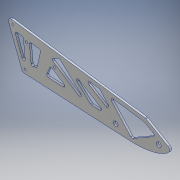
# Autodesk Inventor part: bracket1
Saved by Autodesk Inventor 2018 (Build 220112000, 112)
## iProperties
Created: 2018-03-05
Part Number: bracket1
Material: アルミニウム 6061
Document SubType Name: Modeling
Designer: ku_sk
Density: 2.7 g/cm^3
Appearance: アルミニウム - フラット
Mass: 456.161 g
Surface Area: 733.858 cm^2
Volume: 168.949 cm^3
Author: ku_sk
Autodesk Inventor part; units mm, degrees
ref_plane "YZ Plane" through (0, 0, 0) normal (1, 0, 0) x (0, 1, 0)
ref_plane "XZ Plane" through (0, 0, 0) normal (0, 1, 0) x (-1, 0, 0)
ref_plane "XY Plane" through (0, 0, 0) normal (0, 0, 1) x (1, 0, 0)
sketch "スケッチ2" plane through (0, 0, 0) normal (0, 1, 0) x (-1, 0, 0)
  arc A0 (320.7468, 34.8983) -> (392.1215, 71.6787) centre (243.1623, 273.099) ccw projected
  arc A1 (310.5095, 31.8959) -> (320.7468, 34.8983) centre (264.9264, 206.2785) ccw projected
  arc A2 (290.9118, 29.5172) -> (310.5095, 31.8959) centre (291.9468, 102.9093) ccw projected
  arc A3 (278.6891, 31.4878) -> (290.9118, 29.5172) centre (291.5128, 72.1352) ccw projected
  arc A4 (274.9831, 33.389) -> (278.6891, 31.4878) centre (282.4278, 43.3382) ccw projected
  arc A5 (275.4733, 39.2078) -> (274.9831, 33.389) centre (277.0456, 36.1453) ccw projected
  arc A6 (283.1253, 42.3274) -> (275.4733, 39.2078) centre (297.1464, -3.0086) ccw projected
  arc A7 (310.1184, 49.282) -> (283.1253, 42.3274) centre (369.3413, -236.446) ccw projected
  arc A8 (310.1184, 49.282) -> (326.9533, 52.7997) centre (-771.7798, 5269.0252) ccw projected
  arc A9 (326.9533, 52.7997) -> (357.98, 60.8795) centre (256.8539, 385.5961) ccw projected
  arc A10 (357.98, 60.8795) -> (391.1188, 73.3957) centre (268.9975, 346.6028) ccw projected
  arc A11 (392.1215, 71.6787) -> (391.1188, 73.3957) centre (391.5269, 72.4828) ccw projected
  circle A12 centre (287.1934, 37.1564) radius 3 projected
  circle A13 centre (359.7933, 56.2153) radius 3 projected
  arc A14 (100.5026, -29.4375) -> (303.8176, 17.6729) centre (68.6386, 570.3585) ccw projected
  arc A15 (74.9408, -30.0377) -> (100.5026, -29.4375) centre (77.5861, 401.9345) ccw projected
  arc A16 (28.1912, -23.4013) -> (74.9408, -30.0377) centre (76.0159, 145.5175) ccw projected
  arc A17 (1.2395, -11.312) -> (28.1912, -23.4013) centre (55.8939, 74.446) ccw projected
  arc A18 (-6.0217, -4.7376) -> (1.2395, -11.312) centre (16.9451, 13.3315) ccw projected
  arc A19 (-1.6159, 7.4897) -> (-6.0217, -4.7376) centre (0, 0) ccw projected
  arc A20 (17.9572, 9.9554) -> (-1.6159, 7.4897) centre (22.277, -103.2534) ccw projected
  arc A21 (84.7958, 9.311) -> (17.9572, 9.9554) centre (44.6377, -689.2581) ccw projected
  arc A22 (84.7958, 9.311) -> (126.0099, 7.0084) centre (819.0754, 12782.4716) ccw projected
  arc A23 (126.0099, 7.0084) -> (203.0122, 6.466) centre (170.258, 822.6468) ccw projected
  arc A24 (203.0122, 6.466) -> (303.8176, 17.6729) centre (174.1884, 724.7085) ccw projected
  circle A25 centre (20.0666, -1.5588) radius 5 projected
  circle A26 centre (130.4331, -10.1322) radius 5 projected
  line L0 (100.5026, -29.4375) -> (370, -15.1205)
  line L1 (-3.831, 6.6355) -> (54.1787, 40.1274)
  line L2 (1137.2465, 0) -> (-1089.9509, 0) projected
  line L3 (54.1787, 40.1274) -> (410, 89.8795)
  line L4 (370, -15.1205) -> (410, 89.8795)
  point P0 (0, 0)
  point P1 (371.2778, 57.8193)
  dimension "d7" = 30
  dimension "d115" = 370
  dimension "d164" = 40
  dimension "d165" = 105
  constraints: 8 end point, 2 point on circle, 2 tangent
  measures "d7" angle of L2 L1
  measures "d115" horizontal distance of L0.end point (0, 0)
  measures "d164" horizontal distance of L3.end L0.end
  measures "d165" vertical distance of L0.end L3.end
extrude "押し出し3" add sketch "スケッチ2" along normal blind 5 contours A1 A2 A3 A4 A5 A6 A7 A8 A9 A10 A11 A0 | A15 A16 A17 A18 A19 L2 A25 A14 | A14 L2 L4 L0 | L2 A25 A19 A20 A21 A22 A23 A24 A14 | A14 A24 A23 A22 A21 A20 A19 L1 L3 L4 L2
fillet "フィレット2" radius 6 2 edges at (-54.1787, 2.5, 40.1274) (-370, 2.5, -15.1205)
fillet "フィレット2" radius 7 1 edges at (-410, 2.5, 89.8795)
sketch "スケッチ4" plane through (0, 5, 0) normal (0, 1, 0) x (1, 0, 0)
  circle A0 centre (-362.9716, 5.4798) radius 2.5
  line L0 (-53.1667, -39.5431) -> (3.831, -6.6355) projected
  line L1 (-410, -89.8795) -> (-55.3359, -40.2892) projected
  line L2 (-100.5026, 29.4375) -> (-366.1013, 15.3276) projected
  line L3 (-371.3899, 11.472) -> (-410, -89.8795) projected
  circle A1 centre (-394.6339, -77.6337) radius 2.5
  point P0 (0, 0)
  dimension "d21" = 5
  dimension "d22" = 10
  dimension "d23" = 10
  dimension "d77" = 10
  dimension "d78" = 10
  dimension "d79" = 5
  constraints: 2 centre point
  measures "d21" diameter of A0
  measures "d22" distance from line of L2 A0.centre
  measures "d23" distance from line of L3 A0.centre
  measures "d77" distance from line of A1.centre L1
  measures "d78" distance from line of L3 A1.centre
  measures "d79" diameter of A1
sketch "スケッチ6" plane through (0, 0, 0) normal (0, -1, 0) x (1, 0, 0)
  circle A0 centre (-20.0666, -1.5588) radius 6
  circle A1 centre (-20.0666, -1.5588) radius 5 projected
  circle A2 centre (-130.4331, -10.1322) radius 6
  circle A3 centre (-130.4331, -10.1322) radius 5 projected
  point P0 (0, 0)
  dimension "d29" = 12
  dimension "d30" = 12
  constraints: 2 centre point, 2 concentric
  measures "d29" diameter of A0
  measures "d30" diameter of A2
extrude "押し出し7" cut sketch "スケッチ6" against normal through all
extrude "押し出し9" cut sketch "スケッチ4" against normal through all
sketch "スケッチ10" plane through (0, 0, 0) normal (0, -1, 0) x (1, 0, 0)
  line L0 (-224.8903, 4.737) -> (-291.6748, 48.1758)
  line L1 (-291.3072, 55.0942) -> (-278.1848, 61.7685)
  line L2 (-273.6413, 61.1266) -> (-219.9793, 11.0136)
  line L3 (-195.2115, 1.5663) -> (-230.0713, 34.1207)
  line L4 (-225.2835, 40.4742) -> (-169.1321, 6.7888)
  line L5 (-171.402, -0.6357) -> (-192.6936, 0.4954)
  line L6 (-265.5172, 4.3641) -> (-303.9103, 6.4038)
  line L7 (-307.379, 11.9637) -> (-299.7389, 29.9268)
  line L8 (-293.877, 31.7143) -> (-263.1241, 11.7116)
  line L9 (-370.8987, 15.329) -> (-388.1624, 60.646)
  line L10 (-383.8705, 66.0314) -> (-371.07, 64.2416)
  line L11 (-367.6448, 60.6882) -> (-363.1817, 17.161)
  line L12 (-197.0925, 50.0128) -> (-173.4392, 46.7055)
  line L13 (-171.0224, 45.4227) -> (-149.6481, 21.7177)
  line L14 (-154.6766, 15.609) -> (-199.7042, 42.6212)
  line L15 (-347.6131, 60.9618) -> (-327.0753, 58.0901)
  line L16 (-323.7311, 53.2316) -> (-332.2966, 16.0111)
  line L17 (-335.1019, 13.0603) -> (-342.7409, 10.8908)
  line L18 (-347.8128, 14.3307) -> (-352.1462, 56.5923)
  line L19 (-138.0022, 41.7506) -> (-58.2636, 30.6013)
  line L20 (-56.8175, 30.1039) -> (-33.4921, 16.637)
  line L21 (-33.4921, 9.7088) -> (-86.6743, -20.996)
  line L22 (-91.645, -20.2105) -> (-141.5268, 35.1105)
  line L23 (-53.1667, 39.5431) -> (3.831, 6.6355) projected
  line L24 (-398.2744, 88.24) -> (-55.3359, 40.2892) projected
  line L25 (-371.3899, -11.472) -> (-405.7851, 78.8155) projected
  circle A0 centre (-362.9716, -5.4798) radius 2.5 projected
  circle A1 centre (-394.6339, 77.6337) radius 2.5 projected
  circle A2 centre (-20.0666, -1.5588) radius 6 projected
  circle A3 centre (-130.4331, -10.1322) radius 6 projected
  arc A4 (-398.2744, 88.24) -> (-405.7851, 78.8155) centre (-399.2437, 81.3074) ccw projected
  line L26 (-371.3899, -11.472) -> (-405.7851, 78.8155) projected
  arc A5 (-371.3899, -11.472) -> (-366.1013, -15.3276) centre (-365.783, -9.3361) ccw projected
  line L27 (-100.5026, -29.4375) -> (-366.1013, -15.3276) projected
  arc A6 (-100.5026, -29.4375) -> (-74.9408, -30.0377) centre (-77.5861, 401.9345) ccw projected
  arc A7 (-74.9408, -30.0377) -> (-28.1912, -23.4013) centre (-76.0159, 145.5175) ccw projected
  arc A8 (-28.1912, -23.4013) -> (-1.2395, -11.312) centre (-55.8939, 74.446) ccw projected
  arc A9 (-1.2395, -11.312) -> (6.0217, -4.7376) centre (-16.9451, 13.3315) ccw projected
  arc A10 (6.0217, -4.7376) -> (3.831, 6.6355) centre (0, 0) ccw projected
  line L28 (-53.1667, 39.5431) -> (3.831, 6.6355) projected
  arc A11 (-53.1667, 39.5431) -> (-55.3359, 40.2892) centre (-56.1667, 34.347) ccw projected
  line L29 (-398.2744, 88.24) -> (-55.3359, 40.2892) projected
  circle A12 centre (-287.1934, 37.1564) radius 3 projected
  circle A13 centre (-359.7933, 56.2153) radius 3 projected
  arc A14 (-370.8987, 15.329) -> (-363.1817, 17.161) centre (-367.1608, 16.7529) ccw
  arc A15 (-383.8705, 66.0314) -> (-388.1624, 60.646) centre (-384.4244, 62.07) ccw
  arc A16 (-367.6448, 60.6882) -> (-371.07, 64.2416) centre (-371.6239, 60.2802) ccw
  arc A17 (-347.6131, 60.9618) -> (-352.1462, 56.5923) centre (-348.167, 57.0004) ccw
  arc A18 (-347.8128, 14.3307) -> (-342.7409, 10.8908) centre (-343.8337, 14.7387) ccw
  arc A19 (-335.1019, 13.0603) -> (-332.2966, 16.0111) centre (-336.1947, 16.9081) ccw
  arc A20 (-323.7311, 53.2316) -> (-327.0753, 58.0901) centre (-327.6292, 54.1287) ccw
  arc A21 (-293.877, 31.7143) -> (-299.7389, 29.9268) centre (-296.058, 28.3612) ccw
  arc A22 (-307.379, 11.9637) -> (-303.9103, 6.4038) centre (-303.6981, 10.3981) ccw
  arc A23 (-265.5172, 4.3641) -> (-263.1241, 11.7116) centre (-265.305, 8.3585) ccw
  arc A24 (-291.3072, 55.0942) -> (-291.6748, 48.1758) centre (-289.4938, 51.5289) ccw
  arc A25 (-273.6413, 61.1266) -> (-278.1848, 61.7685) centre (-276.3714, 58.2031) ccw
  arc A26 (-224.8903, 4.737) -> (-219.9793, 11.0136) centre (-222.7094, 8.0901) ccw
  arc A27 (-225.2835, 40.4742) -> (-230.0713, 34.1207) centre (-227.3412, 37.0441) ccw
  arc A28 (-171.402, -0.6357) -> (-169.1321, 6.7888) centre (-171.1898, 3.3587) ccw
  arc A29 (-195.2115, 1.5663) -> (-192.6936, 0.4954) centre (-192.4814, 4.4898) ccw
  arc A30 (-197.0925, 50.0128) -> (-199.7042, 42.6212) centre (-197.6465, 46.0513) ccw
  arc A31 (-171.0224, 45.4227) -> (-173.4392, 46.7055) centre (-173.9931, 42.744) ccw
  arc A32 (-154.6766, 15.609) -> (-149.6481, 21.7177) centre (-152.6188, 19.0391) ccw
  arc A33 (-138.0022, 41.7506) -> (-141.5268, 35.1105) centre (-138.5561, 37.7891) ccw
  arc A34 (-91.645, -20.2105) -> (-86.6743, -20.996) centre (-88.6743, -17.5319) ccw
  arc A35 (-33.4921, 9.7088) -> (-33.4921, 16.637) centre (-35.4921, 13.1729) ccw
  arc A36 (-56.8175, 30.1039) -> (-58.2636, 30.6013) centre (-58.8175, 26.6398) ccw
  point P0 (0, 0)
  point P1 (-186.5641, -20.1916)
  point P2 (-297.4825, 51.9533)
  point P3 (-275.6884, 63.0382)
  point P4 (-194.1474, 0.5726)
  point P5 (-257.6969, 59.9191)
  point P6 (-155.3329, -1.4894)
  point P7 (-250.6102, 3.5722)
  point P8 (-309.6149, 6.7068)
  point P9 (-297.8731, 34.3135)
  point P10 (-360.0825, -13.0636)
  point P11 (-390.5709, 66.9683)
  point P12 (-367.9646, 63.8074)
  point P13 (-216.5638, 52.7353)
  point P14 (-171.9973, 46.5039)
  point P15 (-131.7251, 1.8403)
  point P16 (-352.6667, 61.6684)
  point P17 (-322.7521, 57.4857)
  point P18 (-332.8269, 13.7064)
  point P19 (-347.3266, 9.5885)
  point P20 (-148.8863, 43.2724)
  point P21 (-57.4921, 30.4934)
  point P22 (-27.4921, 13.1729)
  point P23 (-89.4775, -22.6144)
  dimension "d194" = 10
  dimension "d196" = 10
  dimension "d197" = 20
  dimension "d198" = 10
  dimension "d199" = 60
  dimension "d200" = 40
  dimension "d201" = 30
  dimension "d202" = 70
  dimension "d203" = 15
  dimension "d204" = 15
  dimension "d205" = 10
  dimension "d206" = 15
  dimension "d207" = 15
  dimension "d209" = 25
  dimension "d210" = 15
  dimension "d213" = 80
  dimension "d214" = 85
  dimension "d216" = 70
  dimension "d218" = 45
  dimension "d219" = 70
  dimension "d222" = 30
  dimension "d224" = 85
  dimension "d225" = 30
  dimension "d226" = 30
  dimension "d227" = 60
  dimension "d231" = 110
  dimension "d237" = 23
  dimension "d238" = 45
  dimension "d240" = 4
  constraints: 46 end point, 46 point on circle, 46 point on line, 46 tangent, 23 centre point, 22 equal radius, 11 parallel, 3 collinear
  measures "d194" distance between parallel lines of L23 L20
  measures "d196" distance between parallel lines of L24 L19
  measures "d197" distance between parallel lines of L24 L15
  measures "d198" distance between parallel lines of L25 L9
  measures "d199" angle of L21 L20
  measures "d200" angle of L22 L19
  measures "d201" distance from line of point (-57.492, 30.493) L21
  measures "d202" distance from line of point (-27.492, 13.173) L22
  measures "d203" distance between parallel lines of L22 L13
  measures "d204" distance between parallel lines of L4 L14
  measures "d205" distance between parallel lines of L2 L3
  measures "d206" angle of L9 L11
  measures "d207" distance between parallel lines of L8 L0
  measures "d209" distance between parallel lines of L27 L6
  measures "d210" distance between parallel lines of L18 L11
  measures "d213" angle of L18 L17
  measures "d214" angle of L16 L15
  measures "d216" distance from line of L26 point (-322.752, 57.486)
  measures "d218" distance from line of L25 point (-332.827, 13.706)
  measures "d219" angle of L6 L7
  measures "d222" angle of L6 L8
  measures "d224" distance from line of L25 point (-297.873, 34.314)
  measures "d225" distance of point (-309.615, 6.707) point (-297.873, 34.314)
  measures "d226" distance from line of L26 point (-367.965, 63.807)
  measures "d227" angle of L0 L1
  measures "d231" angle of L1 L2
  measures "d237" angle of L14 L12
  measures "d238" distance of point (-216.564, 52.735) point (-171.997, 46.504)
  measures "d240" radius of A14
extrude "押し出し13" cut sketch "スケッチ10" against normal through all contours L0 A24 L1 A25 L2 A26 | L3 A27 L4 A28 L5 A29 | L6 A22 L7 A21 L8 A23 | L9 A15 L10 A16 L11 A14 | L12 A31 L13 A32 L14 A30 | L15 A20 L16 A19 L17 A18 L18 A17 | L19 A36 L20 A35 L21 A34 L22 A33
